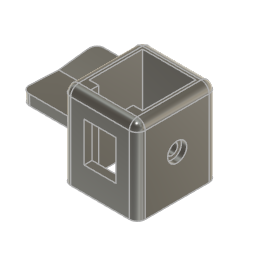
pole_holder_experiment v6 (Autodesk Fusion 360 archive; units mm, degrees)
design "pole_holder_experiment" references "master_params"
Autodesk Fusion 360 part; units mm, degrees
derive "Derived from master_params v0" from "master_params v0"
sketch "Sketch1" plane through (0, 0, 0) normal (0, 0, 1) x (1, 0, 0)
  line L0 (-10.05, -10.05) -> (10.05, -10.05)
  line L1 (10.05, -10.05) -> (10.05, 10.05)
  line L2 (10.05, 10.05) -> (-10.05, 10.05)
  line L3 (-10.05, 10.05) -> (-10.05, -10.05)
  line L4 (-10.05, 10.05) -> (10.05, -10.05) construction
  line L5 (14.05, 14.05) -> (-14.05, 14.05)
  line L6 (-14.05, 14.05) -> (-14.05, -14.05)
  line L7 (-14.05, -14.05) -> (14.05, -14.05)
  line L8 (14.05, -14.05) -> (14.05, 14.05)
  line L9 (14.05, 14.05) -> (-14.05, -14.05) construction
  line L10 (-14.05, 14.05) -> (14.05, -14.05) construction
  line L11 (14.05, 14.05) -> (16.05, 14.05)
  line L12 (16.05, 14.05) -> (16.05, -14.05)
  line L13 (16.05, -14.05) -> (14.05, -14.05)
  line L14 (14.05, -14.05) -> (14.05, 14.05)
  line L15 (-14.05, -14.05) -> (14.05, -14.05)
  line L16 (14.05, -14.05) -> (14.05, -16.05)
  line L17 (14.05, -16.05) -> (-14.05, -16.05)
  line L18 (-14.05, -16.05) -> (-14.05, -14.05)
  constraint horizontal L0
  constraint vertical L1
  constraint horizontal L2
  constraint vertical L3
  constraint midpoint origin L4
  constraint equal L1 L2
  constraint horizontal L5
  constraint perpendicular L5 L6
  constraint parallel L5 L7
  constraint parallel L6 L8
  constraint coincident L9 origin
  constraint coincident L10 origin
  constraint equal L5 L8
  constraint horizontal L11
  constraint vertical L12
  constraint horizontal L13
  constraint vertical L14
  constraint collinear L7 L13
  constraint horizontal L15
  constraint vertical L16
  constraint horizontal L17
  constraint vertical L18
  constraint collinear L8 L16
  measures "d1" distance of L1.end L2.end
  measures "d4" distance of L1 L8
  measures "d38" distance of L12 L14
  measures "d57" distance of L6.end L17.end
extrude "Extrude2" add sketch "Sketch1" along normal blind 50 and the other way blind 200 contours L0 L1 L2 L3 makes body 1
extrude "Extrude1" add sketch "Sketch1" along normal blind 27 and the other way blind 5 separate body contours L5 L6 L7 L8 L14 L15 | L7 L15 L16 L17 L18 makes body 2
sketch "Sketch2" plane through (-14.05, 0, 0) normal (-1, 0, 0) x (0, -1, 0)
  line L0 (-14.05, -5) -> (16.05, -5)
  line L1 (16.05, 27) -> (-14.05, 27)
  line L2 (-14.05, 27) -> (-14.05, -5)
  line L3 (1, 27) -> (0, 0) construction
  line L4 (-13.5871, 12.7593) -> (0.4078, 11.011)
  line L5 (-13.5871, 12.7593) -> (-13.439, 16.7566)
  line L6 (-13.439, 16.7566) -> (0.5559, 15.0082)
  line L7 (0.4078, 11.011) -> (0.5559, 15.0082)
  line L8 (0.4078, 11.011) -> (0.5559, 15.0082)
  line L9 (14.4937, 11.7193) -> (0.4078, 11.011)
  line L10 (14.4937, 11.7193) -> (14.6417, 15.7166)
  line L11 (14.6417, 15.7166) -> (0.5559, 15.0082)
  line L12 (16.05, -5) -> (16.05, 27)
  dimension "d7" = 85
  dimension "d8" = 4
  dimension "d9" = 12
  constraint midpoint L1 L3.start
  constraint coincident L3.end origin
  constraint coincident L3 L4.end
  constraint parallel L3 L5
  constraint coincident L3 L6.end
  constraint parallel L4 L6
  constraint symmetric L3 L4.start L9.start
  constraint symmetric L3 L4.end L7.start
  constraint symmetric L3 L5.end L10.end
  constraint symmetric L3 L6.end L7.end
  measures "d7" angle of L3 L6
  measures "d8" distance of L4.end L6.end
  measures "d9" distance of L3.start L6.end
extrude "Extrude3" add sketch "Sketch2" along normal blind 17 contours L4 L5 L6 L7 L8 | L7 L8 L9 L10 L11 bodies 2
sketch "Sketch7" plane through (0, -16.05, 0) normal (0, -1, 0) x (1, 0, 0)
  line L0 (-14.05, 12.2477) -> (-14.05, 16.2477)
  line L1 (0, 26.4901) -> (0, -5.5099) construction
  line L2 (-6, 4.2193) -> (6, 4.2193)
  line L3 (6, 4.2193) -> (6, 19.2193)
  line L4 (6, 19.2193) -> (-6, 19.2193)
  line L5 (-6, 19.2193) -> (-6, 4.2193)
  line L6 (-14.05, 11.7193) -> (14.05, 11.7193) construction
  line L7 (14.05, -5) -> (14.05, 27)
  line L8 (14.05, 27) -> (-14.05, 27)
  line L9 (-14.05, 27) -> (-14.05, -5)
  line L10 (-14.05, -5) -> (14.05, -5)
  line L11 (-14.05, 11.7193) -> (-31.05, 11.7193)
  dimension "d39" = 15
  dimension "d40" = 12
  constraint horizontal L2
  constraint vertical L3
  constraint horizontal L4
  constraint vertical L5
  constraint symmetric L1 L3.end L4.end
  constraint symmetric L2 L4 L6
  constraint collinear L6 L11
  measures "d39" distance of L2.start L4.end
  measures "d40" distance of L3.end L4.end
extrude "Extrude10" cut sketch "Sketch7" against normal up to surface (6 mm away) contours L2 L3 L4 L5 bodies 2
sketch "Sketch8" plane through (14.05, 0, 0) normal (1, 0, 0) x (0, 1, 0)
  line L0 (14.05, -5) -> (14.05, 27)
  line L1 (14.05, 27) -> (-16.05, 27)
  line L2 (-16.05, -5) -> (14.05, -5)
  line L3 (-1, 27) -> (-1, -5) construction
  line L4 (-16.05, 11) -> (14.05, 11) construction
  circle A0 centre (-1, 11) radius 2.15
  circle A1 centre (-1, 11) radius 3.6
  line L5 (-16.05, 27) -> (-16.05, -5)
  dimension "d45" = 4.3
  dimension "d46" = 7.2
  constraint midpoint L1 L3.start
  constraint midpoint L2 L3.end
  constraint coincident L0 L4.end
  constraint perpendicular L0 L4
  constraint midpoint L4 A0.centre
  constraint concentric A0 A1
  constraint midpoint L3 A0.centre
  measures "d45" diameter of A0
  measures "d46" diameter of A1
extrude "Extrude11" cut sketch "Sketch8" against normal up to surface (4 mm away) contours A0 bodies 2
extrude "Extrude12" cut sketch "Sketch8" against normal blind 2 contours A1 bodies 2
fillet "Fillet2" radius 3 10 edges at (-14.05, -16.05, 11) (-31.05, -14.5677, 13.718) (-31.05, 13.513, 14.758) (-14.05, -1, 27) (-14.05, 14.05, 11) (0, -16.05, 27) (14.05, -16.05, 11) (14.05, -1, 27) (14.05, 14.05, 11) (0, 14.05, 27) on bodies 2
sketch "Sketch9" plane through (0, -14.0404, -0.52) normal (0, -0.999315, -0.037012) x (1, 0, 0)
  line L0 (-28.05, 12.2477) -> (-13.6798, 12.2477)
  line L1 (-13.5929, 16.2477) -> (-28.05, 16.2477)
  line L2 (-13.6798, 12.2477) -> (12.05, 12.2477) construction
  line L3 (-6.0005, 15.1745) -> (-12.0504, 15.1745)
  line L4 (-12.0504, 15.1745) -> (-12.0504, 9.321)
  line L5 (-12.0504, 9.321) -> (-6.0005, 9.321)
  line L6 (-6.0005, 9.321) -> (-6.0005, 15.1745)
  line L7 (6, 15.1745) -> (12.05, 15.1745)
  line L8 (12.05, 15.1745) -> (12.05, 9.321)
  line L9 (12.05, 9.321) -> (6, 9.321)
  line L10 (6, 9.321) -> (6, 15.1745)
  line L11 (-28.05, 16.2477) -> (-28.05, 12.2477)
  ellipse E0 centre (-11.05, -26.7584) end of major axis (-11.05, 54.2971) minor radius 3 (-13.5929, 16.2477) -> (-13.6798, 12.2477) ccw
  point P0 (-13.6798, 12.2477)
  point P1 (-28.05, 12.2477)
  constraint coincident P0 L0.end
  constraint horizontal L3
  constraint vertical L4
  constraint horizontal L5
  constraint vertical L6
  constraint horizontal L7
  constraint vertical L8
  constraint horizontal L9
  constraint vertical L10
  constraint symmetric L2 L3 L5
  constraint collinear L5 L9
  constraint collinear L3 L7
extrude "Extrude13" cut sketch "Sketch9" along normal up to surface contours L3 L4 L5 L6 | L7 L8 L9 L10 end surface through (-10.05, -10.05, 0) normal (0, 1, 0) offset 0 bodies 2
extrude "Extrude14" add sketch "Sketch9" along normal up to surface contours L3 L4 L5 L6 | L7 L8 L9 L10 end surface through (-10.05, -10.05, 0) normal (0, 1, 0) offset 0 bodies 2
sketch "Sketch10" plane through (0, 0, 27) normal (0, 0, 1) x (-1, 0, 0)
  line L0 (10.05, 10.05) -> (10.05, -10.05)
  line L1 (10.05, -10.05) -> (-10.05, -10.05)
  line L2 (-10.05, -10.05) -> (-10.05, 10.05)
  line L3 (-10.05, 10.05) -> (10.05, 10.05)
  line L4 (-11.05, 13.05) -> (-11.05, -11.05)
  line L5 (-11.05, -11.05) -> (11.05, -11.05)
  line L6 (11.05, -11.05) -> (11.05, 13.05)
  line L7 (11.05, 13.05) -> (-11.05, 13.05)
  line L8 (6.5, 10.05) -> (-6.5, 10.05)
  line L9 (-6.5, 10.05) -> (-6.5, 13.05)
  line L10 (-6.5, 13.05) -> (6.5, 13.05)
  line L11 (6.5, 13.05) -> (6.5, 10.05)
  line L12 (0, 0) -> (0, 16.05) construction
  line L13 (11.05, 16.05) -> (-11.05, 16.05)
  dimension "d58" = 3
  dimension "d59" = 13
  constraint horizontal L8
  constraint vertical L9
  constraint horizontal L10
  constraint vertical L11
  constraint coincident L3 L8.start
  constraint coincident L12.start origin
  constraint perpendicular L7 L12
  constraint midpoint L12.end L13
  constraint symmetric L9.end L10.end L12
  measures "d58" distance of L8.end L9.end
  measures "d59" distance of L8.start L8.end
extrude "Extrude15" cut sketch "Sketch10" against normal blind 35 contours L3 L7 L8 L9 L10 L11 bodies 2
ref_plane "WorkPlane1" through (22.05, -1, 9.5) normal (1, 0, 0) x (0, 1, 0)
hidden bodies 1
equation "d1 = 20 mm + aluminum_profile_tolerance_Ref"
equation "pole_diameter_Ref = 18 mm"
equation "aluminum_profile_tolerance_Ref = 0.1 mm"
